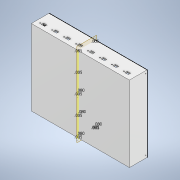
# Autodesk Inventor part: RSA_BOTTOM
Saved by Autodesk Inventor 2020 (Build 240168000, 168)
## iProperties
Created: 2023-03-13
Part Number: RSA_BOTTOM
Material: PC/ABS Plastic
Document SubType Name: Modeling
Designer: catsm
Density: 0.357273 g/cm^3
Appearance: Smooth - White
Author: catsm
Autodesk Inventor part; units mm, degrees
ref_plane "YZ Plane" through (0, 0, 0) normal (1, 0, 0) x (0, 1, 0)
ref_plane "XZ Plane" through (0, 0, 0) normal (0, 1, 0) x (-1, 0, 0)
ref_plane "Work Plane1" through (0, 0, 6.35) normal (0, 0, 1) x (1, 0, 0)
sketch "Sketch1" plane through (0, 0, 6.35) normal (0, 0, 1) x (1, 0, 0)
  line L0 (-137.9455, 29.5421) -> (-136.8665, 29.5421)
  line L1 (-136.8665, 29.5421) -> (-136.8665, 132.2435)
  line L2 (-136.8665, 132.2435) -> (-137.9455, 132.2435)
  line L3 (-137.9455, 132.2435) -> (-137.9455, 29.5421)
  line L4 (-137.9455, 132.2435) -> (117.0456, 132.2435)
  line L5 (117.0456, 132.2435) -> (117.0456, -50.4427)
  line L6 (-137.9455, -50.4427) -> (-137.9455, 132.2435)
  line L7 (117.0456, -50.4427) -> (117.0456, -63.1427)
  line L8 (-137.9455, -50.4427) -> (-137.9455, -63.1427)
  line L9 (-137.9455, -63.1427) -> (117.0456, -63.1427)
  line L10 (-141.7555, 136.0535) -> (120.8556, 136.0535)
  line L11 (120.8556, 136.0535) -> (120.8556, -50.4427)
  line L12 (120.8556, -50.4427) -> (120.8556, -66.9527)
  line L13 (120.8556, -66.9527) -> (-141.7555, -66.9527)
  line L14 (-141.7555, -66.9527) -> (-141.7555, -50.4427)
  line L15 (-141.7555, -50.4427) -> (-141.7555, 136.0535)
  point P0 (0, 0)
  dimension "d143" = 12.7
  dimension "d144" = 12.7
  dimension "d145" = 3.81
  constraints: 32 end point, 4 parallel, 3 perpendicular, 2 horizontal, 2 vertical, 8 other
  measures "d143" distance of L5.end L7.end
  measures "d144" distance of L6.start L8.end
  measures "d145" distance between parallel lines of L6 L15
extrude "Extrusion1" add sketch "Sketch1" along normal blind 3.175 contours L3 L2 L1 L0 | L0 L1 L4 L5 L7 L9 L8 L6 | L10 L11 L12 L13 L14 L15
sketch "Sketch2" plane through (0, 0, 6.35) normal (0, 0, -1) x (-1, 0, 0)
  circle A0 centre (-39.0583, -48.4503) radius 1.016 projected
  circle A1 centre (-115.0583, -48.4503) radius 1.016 projected
  circle A2 centre (-115.0583, -8.4503) radius 1.016 projected
  circle A3 centre (-115.0583, 27.5497) radius 1.016 projected
  circle A4 centre (38.9417, 27.5497) radius 1.016 projected
  circle A5 centre (135.9417, 27.5497) radius 1.016 projected
  circle A6 centre (135.9417, -8.4503) radius 1.016 projected
  circle A7 centre (38.9417, -8.4503) radius 1.016 projected
  circle A8 centre (-39.0583, -8.4503) radius 1.016 projected
  circle A9 centre (-115.1208, 34.2562) radius 1.016 projected
  circle A10 centre (-115.1208, 130.2562) radius 1.016 projected
  circle A11 centre (-89.1208, 130.2562) radius 1.016 projected
  circle A12 centre (-83.1208, 130.2562) radius 1.016 projected
  circle A13 centre (-57.1208, 130.2562) radius 1.016 projected
  circle A14 centre (-51.1208, 130.2562) radius 1.016 projected
  circle A15 centre (-25.1208, 130.2562) radius 1.016 projected
  circle A16 centre (-19.1208, 130.2562) radius 1.016 projected
  circle A17 centre (6.8792, 130.2562) radius 1.016 projected
  circle A18 centre (12.8792, 130.2562) radius 1.016 projected
  circle A19 centre (38.8792, 130.2562) radius 1.016 projected
  circle A20 centre (44.8792, 130.2562) radius 1.016 projected
  circle A21 centre (70.8792, 130.2562) radius 1.016 projected
  circle A22 centre (76.8858, 130.2562) radius 1.016 projected
  circle A23 centre (102.8858, 130.2562) radius 1.016 projected
  circle A24 centre (108.8792, 130.2562) radius 1.016 projected
  circle A25 centre (134.8792, 130.2562) radius 1.016 projected
  circle A26 centre (134.8792, 34.2562) radius 1.016 projected
  circle A27 centre (108.8792, 34.2562) radius 1.016 projected
  circle A28 centre (102.8858, 34.2562) radius 1.016 projected
  circle A29 centre (76.8858, 34.2562) radius 1.016 projected
  circle A30 centre (70.8792, 34.2562) radius 1.016 projected
  circle A31 centre (44.8792, 34.2562) radius 1.016 projected
  circle A32 centre (38.8792, 34.2562) radius 1.016 projected
  circle A33 centre (12.8792, 34.2562) radius 1.016 projected
  circle A34 centre (6.8792, 34.2562) radius 1.016 projected
  circle A35 centre (-19.1208, 34.2562) radius 1.016 projected
  circle A36 centre (-25.1208, 34.2562) radius 1.016 projected
  circle A37 centre (-51.1208, 34.2562) radius 1.016 projected
  circle A38 centre (-57.1208, 34.2562) radius 1.016 projected
  circle A39 centre (-83.1208, 34.2562) radius 1.016 projected
  circle A40 centre (-89.1208, 34.2562) radius 1.016 projected
  circle A41 centre (-115.0583, -48.4503) radius 3.556
  circle A42 centre (-39.0583, -48.4503) radius 3.556
  circle A43 centre (135.9417, -8.4503) radius 3.556
  circle A44 centre (38.9417, -8.4503) radius 3.556
  circle A45 centre (-39.0583, -8.4503) radius 3.556
  circle A46 centre (-115.0583, -8.4503) radius 3.556
  arc A47 (-118.6144, 27.5497) -> (-111.5023, 27.5497) centre (-115.0583, 27.5497) ccw
  arc A48 (-111.5023, 34.2562) -> (-118.6144, 34.2562) centre (-115.0583, 34.2562) ccw
  arc A49 (-89.1208, 37.8122) -> (-89.1208, 30.7002) centre (-89.1208, 34.2562) ccw
  arc A50 (-83.1208, 30.7002) -> (-83.1208, 37.8122) centre (-83.1208, 34.2562) ccw
  arc A51 (-57.1208, 37.8122) -> (-57.1208, 30.7002) centre (-57.1208, 34.2562) ccw
  arc A52 (-51.1208, 30.7002) -> (-51.1208, 37.8122) centre (-51.1208, 34.2562) ccw
  arc A53 (-25.1208, 37.8122) -> (-25.1208, 30.7002) centre (-25.1208, 34.2562) ccw
  arc A54 (-19.1208, 30.7002) -> (-19.1208, 37.8122) centre (-19.1208, 34.2562) ccw
  arc A55 (6.8792, 37.8122) -> (6.8792, 30.7002) centre (6.8792, 34.2562) ccw
  arc A56 (12.8792, 30.7002) -> (12.8792, 37.8122) centre (12.8792, 34.2562) ccw
  arc A57 (38.8792, 37.8122) -> (35.3234, 34.2231) centre (38.8792, 34.2562) ccw
  arc A58 (47.5417, 31.8991) -> (44.8792, 37.8122) centre (44.8792, 34.2562) ccw
  arc A59 (35.3858, 27.5166) -> (41.6041, 25.1925) centre (38.9417, 27.5497) ccw
  circle A60 centre (70.8792, 34.2562) radius 3.556
  circle A61 centre (76.8858, 34.2562) radius 3.556
  arc A62 (102.8858, 37.8122) -> (102.8858, 30.7002) centre (102.8858, 34.2562) ccw
  arc A63 (108.8792, 30.7002) -> (108.8792, 37.8122) centre (108.8792, 34.2562) ccw
  arc A64 (138.3914, 34.8126) -> (131.367, 33.6998) centre (134.8792, 34.2562) ccw
  arc A65 (132.4294, 26.9933) -> (139.4539, 28.1061) centre (135.9417, 27.5497) ccw
  circle A66 centre (134.8792, 130.2562) radius 3.556
  arc A67 (102.8858, 133.8122) -> (102.8858, 126.7002) centre (102.8858, 130.2562) ccw
  arc A68 (76.8858, 126.7002) -> (76.8858, 133.8122) centre (76.8858, 130.2562) ccw
  arc A69 (70.8792, 133.8122) -> (70.8792, 126.7002) centre (70.8792, 130.2562) ccw
  arc A70 (44.8792, 126.7002) -> (44.8792, 133.8122) centre (44.8792, 130.2562) ccw
  arc A71 (38.8792, 133.8122) -> (38.8792, 126.7002) centre (38.8792, 130.2562) ccw
  arc A72 (12.8792, 126.7002) -> (12.8792, 133.8122) centre (12.8792, 130.2562) ccw
  arc A73 (6.8792, 133.8122) -> (6.8792, 126.7002) centre (6.8792, 130.2562) ccw
  arc A74 (-19.1208, 126.7002) -> (-19.1208, 133.8122) centre (-19.1208, 130.2562) ccw
  arc A75 (-25.1208, 133.8122) -> (-25.1208, 126.7002) centre (-25.1208, 130.2562) ccw
  arc A76 (-51.1208, 126.7002) -> (-51.1208, 133.8122) centre (-51.1208, 130.2562) ccw
  arc A77 (-57.1208, 133.8122) -> (-57.1208, 126.7002) centre (-57.1208, 130.2562) ccw
  arc A78 (-83.1208, 126.7002) -> (-83.1208, 133.8122) centre (-83.1208, 130.2562) ccw
  arc A79 (-89.1208, 133.8122) -> (-89.1208, 126.7002) centre (-89.1208, 130.2562) ccw
  circle A80 centre (-115.0583, 130.2562) radius 3.556
  line L0 (131.367, 33.6998) -> (132.4294, 26.9933)
  line L1 (138.3914, 34.8126) -> (139.4539, 28.1061)
  line L2 (108.8792, 37.8122) -> (102.8858, 37.8122)
  line L3 (108.8792, 30.7002) -> (102.8858, 30.7002)
  line L4 (76.8858, 37.8122) -> (70.8792, 37.8122)
  line L5 (76.8858, 30.7002) -> (70.8792, 30.7002)
  line L6 (44.8792, 37.8122) -> (38.8792, 37.8122)
  line L7 (35.3234, 34.2231) -> (35.3858, 27.5166)
  line L8 (41.6041, 25.1925) -> (47.5417, 31.8991)
  line L9 (6.8792, 37.8122) -> (12.8792, 37.8122)
  line L10 (12.8792, 30.7002) -> (6.8792, 30.7002)
  line L11 (-19.1208, 37.8122) -> (-25.1208, 37.8122)
  line L12 (-19.1208, 30.7002) -> (-25.1208, 30.7002)
  line L13 (-51.1208, 37.8122) -> (-57.1208, 37.8122)
  line L14 (-57.1208, 30.7002) -> (-51.1208, 30.7002)
  line L15 (-83.1208, 37.8122) -> (-89.1208, 37.8122)
  line L16 (-89.1208, 30.7002) -> (-83.1208, 30.7002)
  line L17 (-111.5023, 34.2562) -> (-111.5023, 27.5497)
  line L18 (-118.6144, 27.5497) -> (-118.6144, 34.2562)
  line L19 (-89.1208, 133.8122) -> (-83.1208, 133.8122)
  line L20 (-83.1208, 126.7002) -> (-89.1208, 126.7002)
  line L21 (-57.1208, 133.8122) -> (-51.1208, 133.8122)
  line L22 (-51.1208, 126.7002) -> (-57.1208, 126.7002)
  line L23 (-25.1208, 133.8122) -> (-19.1208, 133.8122)
  line L24 (-19.1208, 126.7002) -> (-25.1208, 126.7002)
  line L25 (6.8792, 133.8122) -> (12.8792, 133.8122)
  line L26 (12.8792, 126.7002) -> (6.8792, 126.7002)
  line L27 (38.8792, 133.8122) -> (44.8792, 133.8122)
  line L28 (44.8792, 126.7002) -> (38.8792, 126.7002)
  line L29 (70.8792, 133.8122) -> (76.8858, 133.8122)
  line L30 (76.8858, 126.7002) -> (70.8792, 126.7002)
  line L31 (102.8858, 133.8122) -> (108.8792, 133.8122)
  line L32 (108.8792, 126.7002) -> (102.8858, 126.7002)
  arc A81 (108.8792, 126.7002) -> (108.8792, 133.8122) centre (108.8792, 130.2562) ccw
  point P0 (0, 0)
  dimension "d4" = 2.54
  constraints: 66 end point, 66 point on circle, 42 point on line, 41 centre point, 20 tangent, 1 parallel, 1 vertical, 7 other
  measures "d4" radial gap between concentric circles of A1 A41
ref_plane "Work Plane2" through (-137.9455, -50.4427, 0) normal (0, 0, 1) x (1, 0, 0)
extrude "Extrusion2" add sketch "Sketch2" along normal up to surface (6.35 mm away) from surface at 0 contours A0 | A1 | A2 | A3 | A4 | A5 | A6 | A7 | A8 | A9 | A10 | A11 | A12 | A13 | A14 | A15 | A16 | A17 | A18 | A19 | A20 | A21 | A22 | A23 | A24 | A25 | A26 | A27 | A28 | A29 | A30 | A31 | A32 | A33 | A34 | A35 | A36 | A37 | A38 | A39 | A40 | A41 | A42 | A43 | A44 | A45 | A46 | L18 A48 L17 A47 | L15 A50 L16 A49 | L13 A52 L14 A51 | L11 A54 L12 A53 | L9 A56 L10 A55 | L6 A58 L8 A59 L7 A57 | A60 A61 | L4 A61 A60 | A60 A61 L5 | A61 A60 | A60 A61 | L2 A63 L3 A62 | L1 A65 L0 A64 | A66 | L31 A81 L32 A67 | L30 A69 L29 A68 | L28 A71 L27 A70 | L26 A73 L25 A72 | L24 A75 L23 A74 | L22 A77 L21 A76 | L20 A79 L19 A78 | A80
sketch "Sketch3" plane through (115.0583, 130.2562, 0) normal (0, 0, -1) x (-1, 0, 0)
  circle A0 centre (-0.0624, 0) radius 1.016 projected
  circle A1 centre (25.9376, 0) radius 1.016 projected
  circle A2 centre (31.9376, 0) radius 1.016 projected
  circle A3 centre (57.9376, 0) radius 1.016 projected
  circle A4 centre (63.9376, 0) radius 1.016 projected
  circle A5 centre (89.9376, 0) radius 1.016 projected
  circle A6 centre (95.9376, 0) radius 1.016 projected
  circle A7 centre (121.9376, 0) radius 1.016 projected
  circle A8 centre (127.9376, 0) radius 1.016 projected
  circle A9 centre (153.9376, 0) radius 1.016 projected
  circle A10 centre (159.9376, 0) radius 1.016 projected
  circle A11 centre (185.9376, 0) radius 1.016 projected
  circle A12 centre (191.9442, 0) radius 1.016 projected
  circle A13 centre (217.9442, 0) radius 1.016 projected
  circle A14 centre (223.9376, 0) radius 1.016 projected
  circle A15 centre (249.9376, 0) radius 1.016 projected
  circle A16 centre (249.9376, -96) radius 1.016 projected
  circle A17 centre (223.9376, -96) radius 1.016 projected
  circle A18 centre (217.9442, -96) radius 1.016 projected
  circle A19 centre (191.9442, -96) radius 1.016 projected
  circle A20 centre (185.9376, -96) radius 1.016 projected
  circle A21 centre (159.9376, -96) radius 1.016 projected
  circle A22 centre (153.9376, -96) radius 1.016 projected
  circle A23 centre (127.9376, -96) radius 1.016 projected
  circle A24 centre (121.9376, -96) radius 1.016 projected
  circle A25 centre (95.9376, -96) radius 1.016 projected
  circle A26 centre (89.9376, -96) radius 1.016 projected
  circle A27 centre (63.9376, -96) radius 1.016 projected
  circle A28 centre (57.9376, -96) radius 1.016 projected
  circle A29 centre (31.9376, -96) radius 1.016 projected
  circle A30 centre (25.9376, -96) radius 1.016 projected
  circle A31 centre (-0.0624, -96) radius 1.016 projected
  circle A32 centre (0, -102.7066) radius 1.016 projected
  circle A33 centre (0, -138.7066) radius 1.016 projected
  circle A34 centre (0, -178.7066) radius 1.016 projected
  circle A35 centre (76, -178.7066) radius 1.016 projected
  circle A36 centre (76, -138.7066) radius 1.016 projected
  circle A37 centre (154, -138.7066) radius 1.016 projected
  circle A38 centre (251, -138.7066) radius 1.016 projected
  circle A39 centre (251, -102.7066) radius 1.016 projected
  circle A40 centre (154, -102.7066) radius 1.016 projected
  point P0 (115.0583, -130.2562)
hole "Hole1" at (115.1208, 130.2562, 0) at (89.1208, 130.2562, 0) at (83.1208, 130.2562, 0) at (57.1208, 130.2562, 0) at (51.1208, 130.2562, 0) at (25.1208, 130.2562, 0) at (19.1208, 130.2562, 0) at (-6.8792, 130.2562, 0) at (-12.8792, 130.2562, 0) at (-38.8792, 130.2562, 0) at (-44.8792, 130.2562, 0) at (-70.8792, 130.2562, 0) at (-76.8858, 130.2562, 0) at (-102.8858, 130.2562, 0) at (-108.8792, 130.2562, 0) at (-134.8792, 130.2562, 0) at (-135.9417, 27.5497, 0) at (-134.8792, 34.2562, 0) at (-108.8792, 34.2562, 0) at (-102.8858, 34.2562, 0) at (-76.8858, 34.2562, 0) at (-70.8792, 34.2562, 0) at (-44.8792, 34.2562, 0) at (-38.8792, 34.2562, 0) at (-38.9417, 27.5497, 0) at (-12.8792, 34.2562, 0) at (-6.8792, 34.2562, 0) at (19.1208, 34.2562, 0) at (25.1208, 34.2562, 0) at (51.1208, 34.2562, 0) at (57.1208, 34.2562, 0) at (83.1208, 34.2562, 0) at (89.1208, 34.2562, 0) at (115.1208, 34.2562, 0) at (115.0583, 27.5497, 0) at (-135.9417, -8.4503, 0) at (-38.9417, -8.4503, 0) at (39.0583, -8.4503, 0) at (39.0583, -48.4503, 0) at (115.0583, -48.4503, 0) at (115.0583, -8.4503, 0) direction (0, 0, 1) diameter 3.556 depth 6.35 countersink diameter 3.81 countersink angle 82
sketch "Sketch5" plane through (0, 0, 6.35) normal (0, 0, -1) x (-1, 0, 0)
  line L0 (141.7555, -66.9527) -> (-120.8556, -66.9527) projected
  circle A0 centre (135.9417, -8.4503) radius 3.556 projected
  circle A1 centre (-115.0583, -48.4503) radius 3.556 projected
  circle A2 centre (-39.0583, -8.4503) radius 3.556 projected
  arc A3 (-51.1208, 30.7002) -> (-51.1208, 37.8122) centre (-51.1208, 34.2562) ccw projected
  line L1 (-51.1208, 30.7002) -> (-57.1208, 30.7002) projected
  arc A4 (-57.1208, 37.8122) -> (-57.1208, 30.7002) centre (-57.1208, 34.2562) ccw projected
  line L2 (-57.1208, 37.8122) -> (-51.1208, 37.8122) projected
  line L3 (76.8858, 30.7002) -> (70.8792, 30.7002) projected
  arc A5 (70.8792, 37.8122) -> (70.8792, 30.7002) centre (70.8792, 34.2562) ccw projected
  line L4 (70.8792, 37.8122) -> (76.8858, 37.8122) projected
  arc A6 (76.8858, 30.7002) -> (76.8858, 37.8122) centre (76.8858, 34.2562) ccw projected
  arc A7 (102.8858, 133.8122) -> (102.8858, 126.7002) centre (102.8858, 130.2562) ccw projected
  line L5 (102.8858, 133.8122) -> (108.8792, 133.8122) projected
  arc A8 (108.8792, 126.7002) -> (108.8792, 133.8122) centre (108.8792, 130.2562) ccw projected
  line L6 (108.8792, 126.7002) -> (102.8858, 126.7002) projected
  line L7 (-19.1208, 126.7002) -> (-25.1208, 126.7002) projected
  arc A9 (-25.1208, 133.8122) -> (-25.1208, 126.7002) centre (-25.1208, 130.2562) ccw projected
  line L8 (-25.1208, 133.8122) -> (-19.1208, 133.8122) projected
  arc A10 (-19.1208, 126.7002) -> (-19.1208, 133.8122) centre (-19.1208, 130.2562) ccw projected
  circle A11 centre (-115.0583, 130.2562) radius 3.556 projected
  arc A12 (12.8792, 126.7002) -> (12.8792, 133.8122) centre (12.8792, 130.2562) ccw projected
  line L9 (12.8792, 126.7002) -> (6.8792, 126.7002) projected
  arc A13 (6.8792, 133.8122) -> (6.8792, 126.7002) centre (6.8792, 130.2562) ccw projected
  line L10 (6.8792, 133.8122) -> (12.8792, 133.8122) projected
  circle A14 centre (134.8792, 130.2562) radius 3.556 projected
  arc A15 (47.5417, 31.8991) -> (44.8792, 37.8122) centre (44.8792, 34.2562) ccw projected
  line L11 (47.5417, 31.8991) -> (41.6041, 25.1925) projected
  arc A16 (35.3858, 27.5166) -> (41.6041, 25.1925) centre (38.9417, 27.5497) ccw projected
  line L12 (35.3858, 27.5166) -> (35.3234, 34.2231) projected
  arc A17 (38.8792, 37.8122) -> (35.3234, 34.2231) centre (38.8792, 34.2562) ccw projected
  line L13 (38.8792, 37.8122) -> (44.8792, 37.8122) projected
  line L14 (-89.1208, 37.8122) -> (-83.1208, 37.8122) projected
  arc A18 (-83.1208, 30.7002) -> (-83.1208, 37.8122) centre (-83.1208, 34.2562) ccw projected
  line L15 (-83.1208, 30.7002) -> (-89.1208, 30.7002) projected
  arc A19 (-89.1208, 37.8122) -> (-89.1208, 30.7002) centre (-89.1208, 34.2562) ccw projected
  circle A20 centre (38.9417, -8.4503) radius 3.556 projected
  circle A21 centre (-39.0583, -48.4503) radius 3.556 projected
  circle A22 centre (-115.0583, -8.4503) radius 3.556 projected
  line L16 (-25.1208, 37.8122) -> (-19.1208, 37.8122) projected
  arc A23 (-19.1208, 30.7002) -> (-19.1208, 37.8122) centre (-19.1208, 34.2562) ccw projected
  line L17 (-19.1208, 30.7002) -> (-25.1208, 30.7002) projected
  arc A24 (-25.1208, 37.8122) -> (-25.1208, 30.7002) centre (-25.1208, 34.2562) ccw projected
  line L18 (102.8858, 37.8122) -> (108.8792, 37.8122) projected
  arc A25 (108.8792, 30.7002) -> (108.8792, 37.8122) centre (108.8792, 34.2562) ccw projected
  line L19 (108.8792, 30.7002) -> (102.8858, 30.7002) projected
  arc A26 (102.8858, 37.8122) -> (102.8858, 30.7002) centre (102.8858, 34.2562) ccw projected
  line L20 (76.8858, 126.7002) -> (70.8792, 126.7002) projected
  arc A27 (70.8792, 133.8122) -> (70.8792, 126.7002) centre (70.8792, 130.2562) ccw projected
  line L21 (70.8792, 133.8122) -> (76.8858, 133.8122) projected
  arc A28 (76.8858, 126.7002) -> (76.8858, 133.8122) centre (76.8858, 130.2562) ccw projected
  arc A29 (-51.1208, 126.7002) -> (-51.1208, 133.8122) centre (-51.1208, 130.2562) ccw projected
  line L22 (-51.1208, 126.7002) -> (-57.1208, 126.7002) projected
  arc A30 (-57.1208, 133.8122) -> (-57.1208, 126.7002) centre (-57.1208, 130.2562) ccw projected
  line L23 (-57.1208, 133.8122) -> (-51.1208, 133.8122) projected
  arc A31 (-89.1208, 133.8122) -> (-89.1208, 126.7002) centre (-89.1208, 130.2562) ccw projected
  line L24 (-89.1208, 133.8122) -> (-83.1208, 133.8122) projected
  arc A32 (-83.1208, 126.7002) -> (-83.1208, 133.8122) centre (-83.1208, 130.2562) ccw projected
  line L25 (-83.1208, 126.7002) -> (-89.1208, 126.7002) projected
  line L26 (44.8792, 126.7002) -> (38.8792, 126.7002) projected
  arc A33 (38.8792, 133.8122) -> (38.8792, 126.7002) centre (38.8792, 130.2562) ccw projected
  line L27 (38.8792, 133.8122) -> (44.8792, 133.8122) projected
  arc A34 (44.8792, 126.7002) -> (44.8792, 133.8122) centre (44.8792, 130.2562) ccw projected
  arc A35 (132.4294, 26.9933) -> (139.4539, 28.1061) centre (135.9417, 27.5497) ccw projected
  line L28 (132.4294, 26.9933) -> (131.367, 33.6998) projected
  arc A36 (138.3914, 34.8126) -> (131.367, 33.6998) centre (134.8792, 34.2562) ccw projected
  line L29 (138.3914, 34.8126) -> (139.4539, 28.1061) projected
  line L30 (12.8792, 30.7002) -> (6.8792, 30.7002) projected
  arc A37 (6.8792, 37.8122) -> (6.8792, 30.7002) centre (6.8792, 34.2562) ccw projected
  line L31 (6.8792, 37.8122) -> (12.8792, 37.8122) projected
  arc A38 (12.8792, 30.7002) -> (12.8792, 37.8122) centre (12.8792, 34.2562) ccw projected
  arc A39 (-111.5023, 34.2562) -> (-118.6144, 34.2562) centre (-115.0583, 34.2562) ccw projected
  line L32 (-111.5023, 34.2562) -> (-111.5023, 27.5497) projected
  arc A40 (-118.6144, 27.5497) -> (-111.5023, 27.5497) centre (-115.0583, 27.5497) ccw projected
  line L33 (-118.6144, 27.5497) -> (-118.6144, 34.2562) projected
  line L34 (-120.8556, 136.0535) -> (141.7555, 136.0535) projected
  line L35 (-120.8556, -66.9527) -> (-120.8556, 136.0535) projected
  line L36 (141.7555, -66.9527) -> (-120.8556, -66.9527) projected
  line L37 (141.7555, 136.0535) -> (141.7555, -66.9527) projected
  line L38 (-117.6806, 132.8785) -> (138.5805, 132.8785)
  line L39 (138.5805, 132.8785) -> (138.5805, -63.7777)
  line L40 (138.5805, -63.7777) -> (-117.6806, -63.7777)
  line L41 (-117.6806, -63.7777) -> (-117.6806, 132.8785)
  point P0 (0, 0)
  point P1 (-117.6806, 36.6581)
  point P2 (-117.6806, 127.8544)
  point P3 (-117.6806, 132.6581)
  point P4 (-117.4602, 132.8785)
  point P5 (-112.6565, 132.8785)
  point P6 (-91.5226, 132.8785)
  point P7 (-80.719, 132.8785)
  point P8 (-59.5226, 132.8785)
  point P9 (-48.719, 132.8785)
  point P10 (-27.5226, 132.8785)
  point P11 (-16.719, 132.8785)
  point P12 (4.4774, 132.8785)
  point P13 (15.281, 132.8785)
  point P14 (36.4774, 132.8785)
  point P15 (47.281, 132.8785)
  point P16 (68.4774, 132.8785)
  point P17 (79.2876, 132.8785)
  point P18 (100.484, 132.8785)
  point P19 (111.281, 132.8785)
  point P20 (132.4774, 132.8785)
  point P21 (137.281, 132.8785)
  point P22 (138.5805, 33.6193)
  point P23 (138.5805, 25.166)
  point P24 (138.5805, -6.0666)
  point P25 (138.5805, -10.834)
  point P26 (-117.6806, -50.8521)
  point P27 (-117.6806, -46.0485)
  point P28 (-117.6806, -10.8521)
  point P29 (-117.6806, -6.0485)
  point P30 (-117.6806, 25.1479)
  dimension "d146" = 3.175
  constraints: 8 end point, 3 other
  measures "d146" distance between parallel lines of L35 L41
extrude "Extrusion3" add sketch "Sketch5" along normal blind 44.45 contours L0 L35 L34 L37 | A0 L39 | L39 L29 A35 | A1 L41 | L38 A14 | A22 L41 | L38 A7 L5 A8 | A40 L33 A39 L41 | L38 A27 L21 A28 | A11 L41 | L38 A33 L27 A34 | A11 L38 | L38 A13 L10 A12 | A31 L24 A32 L38 | L38 A9 L8 A10 | A30 L23 A29 L38 picked at (138.8862, -8.4503) picked at (-117.9918, -48.4503) picked at (135.1692, 133.1537) picked at (-117.9918, -8.4503)
sketch "Sketch12" plane through (0, 0, 6.35) normal (0, 0, -1) x (-1, 0, 0)
  line L0 (130.6303, -56.3355) -> (123.8993, -56.3355) construction
  line L1 (130.6303, -54.748) -> (123.8993, -54.748)
  line L2 (123.8993, -57.923) -> (130.6303, -57.923)
  arc A0 (130.6303, -57.923) -> (130.6303, -54.748) centre (130.6303, -56.3355) ccw
  arc A1 (123.8993, -54.748) -> (123.8993, -57.923) centre (123.8993, -56.3355) ccw
  line L3 (-117.6806, -63.7777) -> (138.5805, -63.7777) projected
  point P0 (0, 0)
  point P1 (127.2648, -56.3355)
  dimension "d60" = 1.5875
  dimension "d63" = 6.731
  dimension "d64" = 3.175
  dimension "d160" = 7.4422
  constraints: 8 end point, 4 point on circle, 4 tangent, 2 centre point, 1 horizontal, 1 midpoint, 1 parallel
  measures "d60" radius of A1
  measures "d63" distance of L2.start L2.end
  measures "d64" distance between parallel lines of L1 L2
  measures "d160" distance from line of L3 point (127.265, -56.335)
extrude "Extrusion8" add sketch "Sketch12" along normal blind 6.35
sketch "Sketch25" plane through (-141.7555, 136.0535, 9.525) normal (0, 1, 0) x (1, 0, 0)
  line L0 (24.476, 14.5664) -> (24.476, 11.5165) projected
  line L1 (15.2765, 11.5165) -> (15.2765, 14.5664) projected
  line L2 (34.8636, 11.125) -> (4.889, 11.125) projected
  line L3 (15.2765, 11.125) -> (24.476, 11.125)
  line L4 (24.476, 11.125) -> (24.476, 17.475)
  line L5 (24.476, 17.475) -> (15.2765, 17.475)
  line L6 (15.2765, 17.475) -> (15.2765, 11.125)
  circle A0 centre (11.022, 12.7125) radius 1.5875
  line L7 (56.48, 17.475) -> (47.2805, 17.475)
  line L8 (47.2805, 11.125) -> (56.48, 11.125)
  line L9 (56.48, 11.125) -> (56.48, 17.475)
  line L10 (47.2805, 17.475) -> (47.2805, 11.125)
  circle A1 centre (43.026, 12.7125) radius 1.5875
  line L11 (88.484, 17.475) -> (79.2845, 17.475)
  line L12 (79.2845, 11.125) -> (88.484, 11.125)
  line L13 (88.484, 11.125) -> (88.484, 17.475)
  line L14 (79.2845, 17.475) -> (79.2845, 11.125)
  circle A2 centre (75.03, 12.7125) radius 1.5875
  line L15 (120.488, 17.475) -> (111.2885, 17.475)
  line L16 (111.2885, 11.125) -> (120.488, 11.125)
  line L17 (120.488, 11.125) -> (120.488, 17.475)
  line L18 (111.2885, 17.475) -> (111.2885, 11.125)
  circle A3 centre (107.034, 12.7125) radius 1.5875
  line L19 (152.492, 17.475) -> (143.2925, 17.475)
  line L20 (143.2925, 11.125) -> (152.492, 11.125)
  line L21 (152.492, 11.125) -> (152.492, 17.475)
  line L22 (143.2925, 17.475) -> (143.2925, 11.125)
  circle A4 centre (139.038, 12.7125) radius 1.5875
  line L23 (184.496, 17.475) -> (175.2965, 17.475)
  line L24 (175.2965, 11.125) -> (184.496, 11.125)
  line L25 (184.496, 11.125) -> (184.496, 17.475)
  line L26 (175.2965, 17.475) -> (175.2965, 11.125)
  circle A5 centre (171.042, 12.7125) radius 1.5875
  line L27 (216.5, 17.475) -> (207.3005, 17.475)
  line L28 (207.3005, 11.125) -> (216.5, 11.125)
  line L29 (216.5, 11.125) -> (216.5, 17.475)
  line L30 (207.3005, 17.475) -> (207.3005, 11.125)
  circle A6 centre (203.046, 12.7125) radius 1.5875
  line L31 (248.504, 17.475) -> (239.3045, 17.475)
  line L32 (239.3045, 11.125) -> (248.504, 11.125)
  line L33 (248.504, 11.125) -> (248.504, 17.475)
  line L34 (239.3045, 17.475) -> (239.3045, 11.125)
  circle A7 centre (235.05, 12.7125) radius 1.5875
  point P0 (141.7555, 9.525)
  dimension "d147" = 6.35
  dimension "d148" = 3.175
  dimension "d149" = 1.5875
  dimension "d150" = 4.2545
  dimension "d153" = 32.004
  constraints: 64 end point, 8 centre point, 2 horizontal, 2 parallel, 1 perpendicular, 1 point on line, 70 other
  measures "d147" distance of L4.end L3.end
  measures "d148" diameter of A0
  measures "d149" distance from line of L2 A0.centre
  measures "d150" distance from line of L1 A0.centre
  measures "d153" distance of L4.end L7.start
extrude "Extrusion19" cut sketch "Sketch25" against normal up to surface (3.175 mm away)
sketch "Sketch26" plane through (-141.7555, -66.9527, 9.525) normal (0, -1, 0) x (1, 0, 0)
  line L0 (18.8563, -14.4272) -> (10.1251, -14.4272) projected
  line L1 (18.8563, -14.4272) -> (18.8563, -11.0998) projected
  line L2 (10.1251, -14.4272) -> (10.1251, -11.0998) projected
  line L3 (18.8563, -11.2522) -> (10.1251, -11.2522) projected
  line L4 (18.8563, -14.4272) -> (10.1251, -14.4272)
  line L5 (10.1251, -14.4272) -> (10.1251, -11.2522)
  line L6 (10.1251, -11.2522) -> (18.8563, -11.2522)
  line L7 (18.8563, -11.2522) -> (18.8563, -14.4272)
  line L8 (19.1103, -14.6812) -> (9.8711, -14.6812)
  line L9 (9.8711, -14.6812) -> (9.8711, -10.9982)
  line L10 (9.8711, -10.9982) -> (19.1103, -10.9982)
  line L11 (19.1103, -10.9982) -> (19.1103, -14.6812)
  circle A0 centre (27.2129, -12.8397) radius 2.54
  circle A1 centre (36.7379, -12.8397) radius 2.54
  circle A2 centre (46.3899, -12.8397) radius 3.175
  line L12 (19.1103, -12.8397) -> (20.9077, -12.8397)
  point P0 (141.7555, -9.525)
  point P1 (20.009, -12.8397)
  dimension "d161" = 0.254
  dimension "d162" = 5.08
  dimension "d163" = 5.08
  dimension "d164" = 6.35
  dimension "d165" = 8.1026
  dimension "d166" = 9.525
  dimension "d167" = 9.652
  constraints: 18 end point, 4 parallel, 3 centre point, 3 horizontal alignment, 2 horizontal, 2 midpoint, 2 perpendicular, 3 other
  measures "d161" distance between parallel lines of L7 L11
  measures "d162" diameter of A0
  measures "d163" diameter of A1
  measures "d164" diameter of A2
  measures "d165" distance from line of L11 A0.centre
  measures "d166" distance of A0.centre A1.centre
  measures "d167" distance of A2.centre A1.centre
extrude "Extrusion20" cut sketch "Sketch26" against normal up to surface (3.175 mm away) contours L0 L2 L3 L1 | L8 L9 L10 L11 | A0 | A1 | A2
sketch "Sketch27" plane through (-141.7555, -66.9527, 9.525) normal (0, -1, 0) x (1, 0, 0)
  circle A0 centre (46.3899, -12.8397) radius 3.175 projected
  circle A1 centre (27.2129, -12.8397) radius 2.54 projected
  circle A2 centre (46.3899, -12.8397) radius 3.175 projected
  line L0 (9.8711, -10.9982) -> (19.1103, -10.9982) projected
  line L1 (19.1103, -10.9982) -> (19.1103, -14.6812) projected
  line L2 (19.1103, -14.6812) -> (9.8711, -14.6812) projected
  line L3 (9.8711, -14.6812) -> (9.8711, -10.9982) projected
  circle A3 centre (36.7379, -12.8397) radius 2.54 projected
  line L4 (262.6111, -47.625) -> (262.6111, 0) projected
  line L5 (0, 0) -> (262.6111, 0) projected
  line L6 (0, 0) -> (0, -47.625) projected
  line L7 (262.6111, -47.625) -> (0, -47.625) projected
  line L8 (8.2836, -16.2687) -> (20.6978, -16.2687)
  line L9 (20.6978, -16.2687) -> (20.6978, -9.4107)
  line L10 (20.6978, -9.4107) -> (8.2836, -9.4107)
  line L11 (8.2836, -9.4107) -> (8.2836, -16.2687)
  circle A4 centre (46.3899, -12.8397) radius 5.715
  point P0 (141.7555, -9.525)
  dimension "d170" = 1.5875
  dimension "d171" = 2.54
  constraints: 8 end point, 1 centre point, 3 other
  measures "d170" distance between parallel lines of L2 L8
  measures "d171" radial gap between concentric circles of A0 A4
extrude "Extrusion21" cut sketch "Sketch27" against normal blind 1.5875 contours L0 L1 L2 L3 | L11 L10 L9 L8 | A4
sketch "Sketch28" plane through (120.8556, -66.9527, 9.525) normal (1, 0, 0) x (0, 0, -1)
  circle A0 centre (43.4975, 196.4022) radius 1.905 projected
  circle A1 centre (43.4975, 6.604) radius 1.905 projected
  circle A2 centre (43.4975, 6.604) radius 1.016
  circle A3 centre (43.4975, 196.4022) radius 1.016
  point P0 (9.525, 66.9527)
  dimension "d174" = 2.032
  dimension "d175" = 2.032
  constraints: 2 centre point, 2 coincident
  measures "d174" diameter of A2
  measures "d175" diameter of A3
extrude "Extrusion22" cut sketch "Sketch28" against normal up to surface (262.6111 mm away) contours A2 | A3
ref_plane "Work Plane3" through (-17.2569, -66.9527, 9.525) normal (1, 0, 0) x (0, 0, -1)
sketch "Sketch29" plane through (-17.2569, -66.9527, 9.525) normal (1, 0, 0) x (0, 0, -1)
  line L0 (47.625, 0) -> (0, 0) projected
  line L1 (47.625, 0) -> (47.625, 3.175)
  line L2 (47.625, 203.0062) -> (47.625, 0) projected
  line L3 (0, 0) -> (0, 203.0062) projected
  line L4 (0, 101.5031) -> (47.625, 101.5031)
  line L5 (47.625, 3.175) -> (47.625, 199.8312) projected
  line L6 (47.625, 1.5875) -> (0, 1.5875)
  line L7 (3.175, 3.175) -> (3.175, 0)
  line L8 (3.175, 0) -> (0, 0)
  line L9 (1.5875, 0) -> (1.5875, 1.5875)
  line L10 (47.625, 0) -> (46.0375, 0)
  line L11 (46.0375, 0) -> (46.0375, 3.175)
  line L12 (3.175, 3.175) -> (47.625, 3.175) projected
  circle A0 centre (46.0375, 1.5875) radius 1.016
  circle A1 centre (1.5875, 1.5875) radius 1.016
  circle A2 centre (1.5875, 101.5031) radius 1.016
  line L13 (1.5875, 1.5875) -> (1.5875, 101.5031)
  line L14 (1.5875, 1.5875) -> (1.5875, 101.5031)
  circle A3 centre (1.5875, 51.5453) radius 1.016
  circle A4 centre (46.0375, 201.4187) radius 1.016
  circle A5 centre (1.5875, 201.4187) radius 1.016
  circle A6 centre (1.5875, 151.4609) radius 1.016
  point P0 (9.525, 66.9527)
  point P1 (47.625, 1.5875)
  dimension "d179" = 1.5875
  dimension "d180" = 2.032
  dimension "d181" = 2.032
  dimension "d182" = 2.032
  dimension "d184" = 2.032
  constraints: 20 end point, 8 point on line, 7 centre point, 6 midpoint, 5 perpendicular, 3 symmetric about line, 2 collinear, 1 coincident, 1 vertical, 3 other
  measures "d179" distance of L0.start L10.end
  measures "d180" diameter of A0
  measures "d181" diameter of A1
  measures "d182" diameter of A2
  measures "d184" diameter of A3
sketch "Sketch30" plane through (-17.2569, -66.9527, 9.525) normal (1, 0, 0) x (0, 0, -1)
  circle A0 centre (1.5875, 1.5875) radius 1.016 projected
  circle A1 centre (46.0375, 1.5875) radius 1.016 projected
  circle A2 centre (1.5875, 51.5453) radius 1.016 projected
  circle A3 centre (1.5875, 101.5031) radius 1.016 projected
  circle A4 centre (1.5875, 151.4609) radius 1.016 projected
  circle A5 centre (1.5875, 201.4187) radius 1.016 projected
  circle A6 centre (46.0375, 201.4187) radius 1.016 projected
  circle A7 centre (46.0375, 201.4187) radius 1.143
  circle A8 centre (1.5875, 201.4187) radius 1.143
  circle A9 centre (1.5875, 151.4609) radius 1.143
  circle A10 centre (1.5875, 101.5031) radius 1.143
  circle A11 centre (1.5875, 51.5453) radius 1.143
  circle A12 centre (1.5875, 1.5875) radius 1.143
  circle A13 centre (46.0375, 1.5875) radius 1.143
  point P0 (9.525, 66.9527)
  dimension "d186" = 0.127
  dimension "d187" = 0.127
  dimension "d188" = 0.127
  dimension "d189" = 0.127
  dimension "d190" = 0.127
  dimension "d191" = 0.127
  dimension "d192" = 0.127
  constraints: 7 centre point
  measures "d186" radial gap between concentric circles of A6 A7
  measures "d187" radial gap between concentric circles of A5 A8
  measures "d188" radial gap between concentric circles of A4 A9
  measures "d189" radial gap between concentric circles of A3 A10
  measures "d190" radial gap between concentric circles of A2 A11
  measures "d191" radial gap between concentric circles of A0 A12
  measures "d192" radial gap between concentric circles of A1 A13
sketch "Sketch31" plane through (0, 0, -38.1) normal (0, 0, -1) x (-1, 0, 0)
  line L0 (17.2569, 136.0535) -> (17.2569, -66.9527) projected
  line L1 (-120.8556, -66.9527) -> (-120.8556, 136.0535) projected
  line L2 (-120.8556, 136.0535) -> (17.2569, 136.0535)
  line L3 (17.2569, 136.0535) -> (17.2569, -66.9527)
  line L4 (17.2569, -66.9527) -> (-120.8556, -66.9527)
  line L5 (-120.8556, -66.9527) -> (-120.8556, 136.0535)
  line L6 (-120.8556, 136.0535) -> (141.7555, 136.0535) projected
  line L7 (141.7555, 136.0535) -> (17.2569, 136.0535)
  line L8 (17.2569, 136.0535) -> (17.2569, -66.9527)
  line L9 (17.2569, -66.9527) -> (141.7555, -66.9527)
  line L10 (141.7555, -66.9527) -> (141.7555, 136.0535)
  point P0 (0, 0)
  constraints: 16 end point, 4 parallel, 2 horizontal, 2 perpendicular
body "Solid1"
